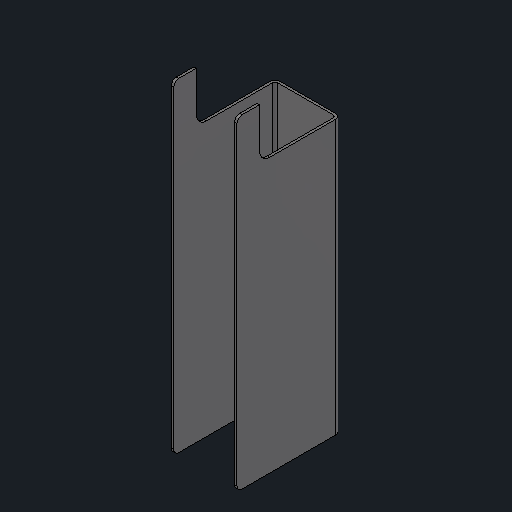
# Autodesk Inventor part: Model-1_Base Tube-2
Saved by Autodesk Inventor 2025.1 (Build 291241000, 241)
## iProperties
RuleStatus: InUse
Created: 2026-02-13
Part Number: Model-1_Base Tube-2
User Status: Released
Material: SS304
Description: Model-1 Base Tube-1
Document SubType Name: Sheet Metal
Designer: Desktop -24
Density: 7.99949 g/cm^3
Appearance: Semi-Polished(1)
Sheet Metal Rule: Default
AfterDocNew0: Mat. Selection
encoded128: ÌStandard Î
encoded39: *STANDARD*
Family: SS304
Author: Desktop -24
Revision Number: 0
Autodesk Inventor part; units mm, degrees
ref_plane "YZ Plane" through (0, 0, 0) normal (1, 0, 0) x (0, 1, 0)
ref_plane "XZ Plane" through (0, 0, 0) normal (0, 1, 0) x (-1, 0, 0)
ref_plane "XY Plane" through (0, 0, 0) normal (0, 0, 1) x (1, 0, 0)
sketch "Sketch7" plane through (0, 0, 0) normal (0, 1, 0) x (-1, 0, 0)
  line L0 (38.1, 0) -> (-38.1, 0)
  line L1 (38.1, 0) -> (38.1, 127)
  line L2 (-38.1, 0) -> (-38.1, 127)
  point P0 (0, 0)
  point P1 (0, 0)
  dimension "d18" = 76.2
  dimension "d19" = 127
  measures "d18" distance of L0.start L0.end
  measures "d19" distance of L0.start L1.end
contour flange "Contour Flange1" sketch "Sketch7" thickness 3.048 bend radius 3.048 width 406.4 along (0, 1, 0) mid plane no both sides no wall seen from (-38.1, 0, 63.5) lies toward (-1, 0, 0) curves L1 L0 L2
bend "Bend1"
corner "Corner1"
sketch "Sketch8" plane through (0, 0, 0) normal (1, 0, 0) x (0, 1, 0)
  line L0 (0, -3.048) -> (406.4, -3.048) projected
  line L1 (406.4, -3.048) -> (342.9, -3.048)
  line L2 (342.9, -3.048) -> (342.9, 98.552)
  line L3 (342.9, 98.552) -> (406.4, 98.552)
  line L4 (406.4, 98.552) -> (406.4, -3.048)
  point P0 (0, 0)
  point P1 (342.9, -3.048)
  dimension "d31" = 101.6
  dimension "d32" = 63.5
  constraints: 8 end point, 2 parallel, 1 horizontal, 1 perpendicular
  measures "d31" distance of L3.end L0.end
  measures "d32" distance between parallel lines of L4 L2
extrude "Cut1" cut sketch "Sketch8" along normal through all both and the other way through all
fillet "Corner Round1" radius 6.35 4 edges at (-39.624, 406.4, 127) (39.624, 406.4, 127) (39.624, 0, 127) (-39.624, 0, 127)
fillet "Corner Round2" radius 12.7 2 edges at (39.624, 342.9, 98.552) (-39.624, 342.9, 98.552)
equation "\"d33\" = Thickness"
equation "\"d20\" = Thickness"
equation "\"d21\" = BendReliefWidth"
equation "\"d22\" = BendReliefDepth"
equation "\"d23\" = MinimumRemnant"
equation "\"d24\" = TransitionRadius"
equation "\"d26\" = BendRadius"
equation "\"d28\" = CornerReliefSize"
equation "\"d29\" = GapSize"
equation "\"d30\" = JacobiRadiusSize"
equation "\"BendRadius\" = Thickness"
equation "\"BendReliefWidth\" = Thickness"
equation "\"BendReliefDepth\" = 0.5 * Thickness"
equation "\"CornerReliefSize\" = 4 * Thickness"
equation "\"MinimumRemnant\" = 2 * Thickness"
equation "\"TransitionRadius\" = BendRadius"
equation "\"JacobiRadiusSize\" = BendRadius"
equation "\"GapSize\" = Thickness"
equation "\"Thickness\" = 3.048"
body "Solid5"
